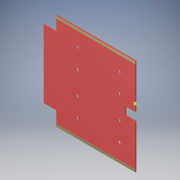
# Autodesk Inventor part: EPS_PCB
Saved by Autodesk Inventor 2018 (Build 220112000, 112)
## iProperties
Created: 2018-01-15
Part Number: EPS_PCB
Material: Epoxy Resin
Document SubType Name: Modeling
Designer: Bradley
Density: 1.14 g/cm^3
Appearance: Smooth - Red
Author: Bradley
Revision Number: 3
Autodesk Inventor part; units mm, degrees
ref_plane "YZ Plane" through (0, 0, 0) normal (1, 0, 0) x (0, 1, 0)
ref_plane "XZ Plane" through (0, 0, 0) normal (0, 1, 0) x (-1, 0, 0)
ref_plane "XY Plane" through (0, 0, 0) normal (0, 0, 1) x (1, 0, 0)
sketch "Sketch1" plane through (0, 0, 0) normal (0, 0, 1) x (1, 0, 0)
  line L0 (0, 33.8) -> (12.5, 33.8)
  line L1 (12.5, 33.8) -> (12.5, 47.9)
  line L2 (12.5, 47.9) -> (91.4, 47.9)
  line L3 (91.4, 47.9) -> (91.4, -47.9)
  line L4 (91.4, -47.9) -> (12.5, -47.9)
  line L5 (12.5, -47.9) -> (12.5, -33.8)
  line L6 (12.5, -33.8) -> (0, -33.8)
  line L7 (0, -33.8) -> (0, 33.8)
  line L8 (-4.5, 48) -> (91.5, 48) construction
  line L9 (91.5, 48) -> (91.5, -48) construction
  line L10 (91.5, -48) -> (-4.5, -48) construction
  line L11 (-4.5, -48) -> (-4.5, 48) construction
  line L12 (-4.4, 47.9) -> (-3.4, 47.9) construction
  line L13 (-3.4, 47.9) -> (-3.4, -47.9) construction
  line L14 (-3.4, -47.9) -> (-4.4, -47.9) construction
  line L15 (-4.4, -47.9) -> (-4.4, 47.9) construction
  point P0 (0, 0)
  point P1 (0, 0)
  point P2 (-4.5, 0)
  dimension "d0" = 67.6
  dimension "d1" = 95.8
  dimension "d2" = 91.4
  dimension "d3" = 12.5
  dimension "d20" = 96
  dimension "d21" = 96
  dimension "d22" = 0.1
  dimension "d23" = 0.1
  dimension "d24" = 1
  dimension "d25" = 0.1
  dimension "d26" = 3.4
  constraints: 32 end point, 8 perpendicular, 4 parallel, 3 collinear, 3 horizontal, 2 midpoint, 2 point on line, 1 coincident, 1 horizontal alignment
  measures "d0" distance of L6.end L0.start
  measures "d1" distance of L2.end L3.end
  measures "d2" distance between parallel lines of L7 L3
  measures "d3" distance of L0.start L0.end
  measures "d20" distance of L8.start L8.end
  measures "d21" distance of L10.end L8.start
  measures "d22" distance between parallel lines of L2 L8
  measures "d23" distance between parallel lines of L9 L3
  measures "d24" distance between parallel lines of L15 L13
  measures "d25" distance between parallel lines of L15 L11
  measures "d26" distance between parallel lines of L7 L13
extrude "Extrusion1" add sketch "Sketch1" along normal mid plane 1
sketch "Sketch2" plane through (0, 0, 0.5) normal (0, 0, 1) x (1, 0, 0)
  line L0 (12.5, 33.8) -> (0, 33.8) projected
  line L1 (0, 33.8) -> (0, -33.8) projected
  line L2 (0, -33.8) -> (12.5, -33.8) projected
  line L3 (12.5, -33.8) -> (12.5, -47.9) projected
  line L4 (12.5, -47.9) -> (91.4, -47.9) projected
  line L5 (91.4, -47.9) -> (91.4, 47.9) projected
  line L6 (91.4, 47.9) -> (12.5, 47.9) projected
  line L7 (12.5, 47.9) -> (12.5, 33.8) projected
  line L8 (91.4, -47.9) -> (91.4, 47.9) projected
  line L9 (12.5, 47.9) -> (91.4, 47.9)
  line L10 (91.4, 47.9) -> (91.4, 45.4)
  line L11 (91.4, 45.4) -> (12.5, 45.4)
  line L12 (12.5, 45.4) -> (12.5, 47.9)
  line L13 (91.4, -47.9) -> (12.5, -47.9)
  line L14 (12.5, -47.9) -> (12.5, -45.4)
  line L15 (12.5, -45.4) -> (91.4, -45.4)
  line L16 (91.4, -45.4) -> (91.4, -47.9)
  point P0 (0, 0)
  dimension "d6" = 2.5
  dimension "d27" = 90.8
  constraints: 16 end point, 4 parallel, 2 horizontal, 2 perpendicular, 2 point on line, 1 collinear
  measures "d6" distance between parallel lines of L4 L15
  measures "d27" distance between parallel lines of L15 L11
extrude "Extrusion2" add sketch "Sketch2" along normal blind 0.1 contours L7 L6 L5 L11 | L5 L4 L3 L15
mirror "Mirror1" about plane through (0, 0, 0) normal (0, 0, 1) of "Extrusion2"
sketch "Sketch3" plane through (0, 0, 0.5) normal (0, 0, 1) x (1, 0, 0)
  circle A0 centre (6, 31.8) radius 0.9
  circle A1 centre (6, -31.8) radius 0.9
  point P0 (0, 0)
  dimension "d9" = 1.8
  dimension "d10" = 6
  dimension "d11" = 31.8
  dimension "d12" = 31.8
  constraints: 2 centre point, 1 equal radius, 1 vertical alignment
  measures "d9" diameter of A0
  measures "d10" horizontal distance of point (0, 0) A0.centre
  measures "d11" vertical distance of point (0, 0) A0.centre
  measures "d12" vertical distance of A1.centre point (0, 0)
extrude "Extrusion3" cut sketch "Sketch3" against normal through all
sketch "Sketch4" plane through (0, 0, 0.5) normal (0, 0, 1) x (1, 0, 0)
  circle A0 centre (6, 31.8) radius 0.9 projected
  circle A1 centre (6, -31.8) radius 0.9 projected
  line L0 (12.5, -45.4) -> (91.4, -45.4) projected
  line L1 (91.4, -45.4) -> (91.4, 45.4) projected
  line L2 (91.4, 45.4) -> (12.5, 45.4) projected
  line L3 (12.5, 45.4) -> (12.5, 33.8) projected
  line L4 (12.5, 33.8) -> (0, 33.8) projected
  line L5 (0, 33.8) -> (0, -33.8) projected
  line L6 (0, -33.8) -> (12.5, -33.8) projected
  line L7 (12.5, -33.8) -> (12.5, -45.4) projected
  line L8 (0, 18.95) -> (3.5, 18.95)
  arc A2 (3.5, 17.95) -> (3.5, 18.95) centre (3.5, 18.45) ccw
  line L9 (3.5, 17.95) -> (0, 17.95)
  point P0 (0, 0)
  dimension "d15" = 17.95
  dimension "d16" = 3.5
  dimension "d17" = 1
  constraints: 4 end point, 2 point on circle, 2 point on line, 2 tangent, 1 centre point, 1 horizontal, 1 perpendicular
  measures "d15" distance from line of point (0, 0) L9
  measures "d16" distance from line of A2.centre L5
  measures "d17" distance between parallel lines of L9 L8
extrude "Extrusion4" cut sketch "Sketch4" against normal through all contours L5 L8 A2 L9
sketch "Sketch5" plane through (0, 0, 0.5) normal (0, 0, 1) x (1, 0, 0)
  line L0 (89.1, 6.3) -> (89.1, -6.3) construction
  line L1 (91.4, -45.4) -> (91.4, 45.4) projected
  line L2 (0, 17.95) -> (0, -33.8) projected
  point P0 (0, 0)
  point P1 (89.1, 0)
  point P2 (91.4, 0)
  dimension "d29" = 12.6
  dimension "d69" = 89.1
  constraints: 2 coincident, 2 end point, 2 midpoint, 1 horizontal alignment, 1 vertical
  measures "d29" distance of L0.start L0.end
  measures "d69" distance between parallel lines of L0 L2
hole "Hole1" at (89.1, 6.3, 0.5) at (89.1, -6.3, 0.5) direction (0, 0, -1) diameter 2.2 end through all clearance for "Socket Head Cap Screw" size "M2" standard "Ansi Metric M Profile"
sketch "Sketch6" plane through (0, 0, 0.5) normal (0, 0, 1) x (1, 0, 0)
  circle A0 centre (89.1, 6.3) radius 1.1 projected
  circle A1 centre (89.1, -6.3) radius 1.1 projected
  line L0 (0, 18.95) -> (3.5, 18.95) projected
  arc A2 (3.5, 17.95) -> (3.5, 18.95) centre (3.5, 18.45) ccw projected
  line L1 (3.5, 17.95) -> (0, 17.95) projected
  line L2 (0, 17.95) -> (0, -33.8) projected
  line L3 (0, -33.8) -> (12.5, -33.8) projected
  line L4 (12.5, -33.8) -> (12.5, -45.4) projected
  line L5 (12.5, -45.4) -> (91.4, -45.4) projected
  line L6 (91.4, -45.4) -> (91.4, 45.4) projected
  line L7 (91.4, 45.4) -> (12.5, 45.4) projected
  line L8 (12.5, 45.4) -> (12.5, 33.8) projected
  line L9 (12.5, 33.8) -> (0, 33.8) projected
  line L10 (0, 33.8) -> (0, 18.95) projected
  circle A3 centre (6, -31.8) radius 0.9 projected
  circle A4 centre (6, 31.8) radius 0.9 projected
  line L11 (91.4, 45.4) -> (91.4, -45.4) projected
  line L12 (91.4, 4) -> (82.4, 4)
  arc A5 (82.4, 4) -> (81.4, 3) centre (82.4, 3) ccw
  line L13 (81.4, 3) -> (81.4, -3)
  arc A6 (81.4, -3) -> (82.4, -4) centre (82.4, -3) ccw
  line L14 (82.4, -4) -> (91.4, -4)
  circle A7 centre (90.7, 11.7) radius 0.7 construction
  circle A8 centre (90.7, 10.3) radius 0.7 construction
  line L15 (91.4, 12.5) -> (90.9, 12.5)
  arc A9 (90.9, 12.5) -> (89.9, 11.5) centre (90.9, 11.5) ccw
  line L16 (89.9, 11.5) -> (89.9, 10.5)
  arc A10 (89.9, 10.5) -> (90.9, 9.5) centre (90.9, 10.5) ccw
  line L17 (90.9, 9.5) -> (91.4, 9.5)
  line L18 (91.4, -45.4) -> (91.4, 45.4) construction
  line L19 (89.9, 11) -> (91.4, 11) construction
  point P0 (0, 0)
  point P1 (81.4, 0)
  dimension "d37" = 1
  dimension "d38" = 8
  dimension "d39" = 1.2
  dimension "d40" = 10
  dimension "d65" = 1.4
  dimension "d66" = 1.5
  dimension "d67" = 3
  dimension "d68" = 11
  constraints: 14 end point, 12 tangent, 8 point on circle, 7 perpendicular, 6 centre point, 5 point on line, 3 equal radius, 2 midpoint, 1 horizontal alignment, 1 parallel
  measures "d37" radius of A5
  measures "d38" distance between parallel lines of L14 L12
  measures "d39" distance edge to line of A0 L12
  measures "d40" distance between parallel lines of L6 L13
  measures "d65" diameter of A7
  measures "d66" distance between parallel lines of L6 L16
  measures "d67" distance between parallel lines of L17 L15
  measures "d68" distance from line of point (0, 0) L19
extrude "Extrusion5" cut sketch "Sketch6" against normal through all contours L6 L17 A10 L16 A9 L15 | L6 L14 A6 L13 A5 L12
sketch "Sketch7" plane through (0, 0, 0.5) normal (0, 0, 1) x (1, 0, 0)
  line L0 (80.65, 7.93) -> (84.65, 7.93) construction
  line L1 (91.4, 4) -> (91.4, 45.4) projected
  point P0 (0, 0)
  dimension "d43" = 7.93
  dimension "d44" = 6.75
  dimension "d45" = 4
  constraints: 2 coincident, 2 end point, 1 horizontal
  measures "d43" distance from line of point (0, 0) L0
  measures "d44" distance from line of L1 L0.end
  measures "d45" distance of L0.start L0.end
hole "Hole2" at (80.65, 7.93, 0.5) at (84.65, 7.93, 0.5) direction (0, 0, -1) diameter 1.7 end through all
fillet "Fillet1" radius 0.5 6 edges at (12.5, -33.8, 0) (12.5, 33.8, 0) (91.4, 4, 0) (91.4, -4, 0) (91.4, 9.5, 0) (91.4, 12.5, 0)
sketch "Sketch8" plane through (0, 0, 0.5) normal (0, 0, 1) x (1, 0, 0)
  arc A0 (91.4, -4.5) -> (90.9, -4) centre (90.9, -4.5) ccw projected
  line L0 (90.9, -4) -> (82.4, -4) projected
  arc A1 (81.4, -3) -> (82.4, -4) centre (82.4, -3) ccw projected
  line L1 (81.4, -3) -> (81.4, 3) projected
  arc A2 (82.4, 4) -> (81.4, 3) centre (82.4, 3) ccw projected
  line L2 (82.4, 4) -> (90.9, 4) projected
  arc A3 (90.9, 4) -> (91.4, 4.5) centre (90.9, 4.5) ccw projected
  line L3 (91.4, 4.5) -> (91.4, 9) projected
  line L4 (91.4, 45.4) -> (12.5, 45.4) projected
  line L5 (12.5, 45.4) -> (12.5, 34.3) projected
  arc A4 (12, 33.8) -> (12.5, 34.3) centre (12, 34.3) ccw projected
  line L6 (12, 33.8) -> (0, 33.8) projected
  line L7 (0, 33.8) -> (0, 18.95) projected
  line L8 (0, 18.95) -> (3.5, 18.95) projected
  arc A5 (3.5, 17.95) -> (3.5, 18.95) centre (3.5, 18.45) ccw projected
  line L9 (3.5, 17.95) -> (0, 17.95) projected
  line L10 (0, 17.95) -> (0, -33.8) projected
  line L11 (0, -33.8) -> (12, -33.8) projected
  arc A6 (12.5, -34.3) -> (12, -33.8) centre (12, -34.3) ccw projected
  line L12 (12.5, -34.3) -> (12.5, -45.4) projected
  line L13 (12.5, -45.4) -> (91.4, -45.4) projected
  line L14 (91.4, -45.4) -> (91.4, -4.5) projected
  circle A7 centre (80.65, 7.93) radius 0.85 projected
  circle A8 centre (84.65, 7.93) radius 0.85 projected
  circle A9 centre (6, 31.8) radius 0.9 projected
  circle A10 centre (6, -31.8) radius 0.9 projected
  circle A11 centre (89.1, -6.3) radius 1.1 projected
  circle A12 centre (89.1, 6.3) radius 1.1 projected
  line L15 (33, 11.5) -> (33, 30.5) construction
  line L16 (75, 30.5) -> (75, 11.5) construction
  line L17 (33, -11.5) -> (33, -30.5) construction
  line L18 (75, -11.5) -> (75, -30.5) construction
  line L19 (0, 0) -> (81.4, 0) construction
  arc A13 (89.9, 10.5) -> (90.9, 9.5) centre (90.9, 10.5) ccw projected
  line L20 (89.9, 10.5) -> (89.9, 11.5) projected
  arc A14 (90.9, 12.5) -> (89.9, 11.5) centre (90.9, 11.5) ccw projected
  line L21 (91.4, 13) -> (91.4, 45.4) projected
  arc A15 (90.9, 12.5) -> (91.4, 13) centre (90.9, 13) ccw projected
  arc A16 (91.4, 9) -> (90.9, 9.5) centre (90.9, 9) ccw projected
  point P0 (33, 21)
  point P1 (75, 21)
  point P2 (75, -21)
  point P3 (33, -21)
  dimension "d54" = 21
  dimension "d55" = 33
  dimension "d56" = 75
  dimension "d57" = 19
  constraints: 10 end point, 8 coincident, 5 midpoint, 4 vertical, 3 symmetric about line, 2 horizontal alignment, 1 parallel
  measures "d54" vertical distance of point (33, -21) L19.start
  measures "d55" distance between parallel lines of L17 L10
  measures "d56" distance between parallel lines of L18 L10
  measures "d57" distance of L17.start L17.end
hole "Hole3" at (33, 30.5, 0.5) at (33, 11.5, 0.5) at (75, 11.5, 0.5) at (75, 30.5, 0.5) at (75, -11.5, 0.5) at (75, -30.5, 0.5) at (33, -30.5, 0.5) at (33, -11.5, 0.5) direction (0, 0, -1) diameter 3 end through all
equation "\"d23\" = d22"
equation "\"d25\" = d22"
equation "\"d12\" = d11"
body "Solid1"
